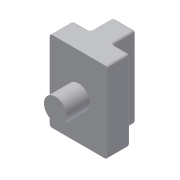
# Autodesk Inventor part: Part3
Saved by Autodesk Inventor 2014 (Build 180170000, 170)
## iProperties
Created: 2013-07-16
Part Number: Part3
Material: Generic
Document SubType Name: Modeling
Density: 1 g/cm^3
Appearance: Default
Autodesk Inventor part; units mm, degrees
ref_plane "YZ Plane" through (0, 0, 0) normal (1, 0, 0) x (0, 1, 0)
ref_plane "XZ Plane" through (0, 0, 0) normal (0, 1, 0) x (-1, 0, 0)
ref_plane "XY Plane" through (0, 0, 0) normal (0, 0, 1) x (1, 0, 0)
sketch "Sketch1" plane through (0, 0, 0) normal (0, 0, 1) x (1, 0, 0)
  line L0 (-25, 0) -> (25, 0)
  line L1 (25, 0) -> (25, 20)
  line L2 (25, 20) -> (10, 20)
  line L3 (10, 20) -> (10, 40)
  line L4 (10, 40) -> (-10, 40)
  line L5 (-10, 40) -> (-10, 20)
  line L6 (-10, 20) -> (-25, 20)
  line L7 (-25, 20) -> (-25, 0)
  line L8 (0, 0) -> (0, 36.7011) construction
  dimension "d0" = 50
  dimension "d1" = 20
  dimension "d2" = 20
  dimension "d3" = 20
  constraints: 18 end point, 6 parallel, 2 perpendicular, 1 collinear, 1 horizontal, 1 midpoint, 2 other
  measures "d0" distance between parallel lines of L1 L7
  measures "d1" distance of L6.end L0.start
  measures "d2" distance of L4.end L5.end
  measures "d3" distance of L3.end L4.end
extrude "Extrusion1" add sketch "Sketch1" along normal mid plane 70
sketch "Sketch2" plane through (-25, 0, 35) normal (0, -1, 0) x (1, 0, 0)
  circle A0 centre (25, -35) radius 10
  dimension "d6" = 20
  constraints: 1 centre point, 1 coincident
  measures "d6" diameter of A0
extrude "Extrusion2" add sketch "Sketch2" along normal blind 20
fillet "Fillet1" radius 2 10 edges at (-10, 40, 0) (-10, 30, 35) (0, 40, 35) (10, 30, 35) (10, 40, 0) (0, 40, -35) (-10, 30, -35) (10, 30, -35) (17.5, 20, 35) (25, 10, 35)
fillet "Fillet1" radius 2 10 edges at (25, 20, 0) (25, 10, -35) (17.5, 20, -35) (10, 20, 0) (-17.5, 20, -35) (-25, 10, -35) (-25, 20, 0) (-10, 20, 0) (-17.5, 20, 35) (-25, 10, 35)
body "Solid1"
